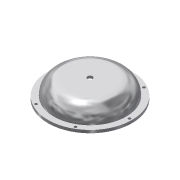
# Autodesk Inventor part: Kugel_oben_V5_Riza
Saved by Autodesk Inventor 2015 (Build 190159000, 159)
## iProperties
Created: 2015-06-19
Part Number: Kugel_oben_V5_Riza
Material: ABS-Kunststoff
Document SubType Name: Modeling
Designer: Johann
Density: 1.06 g/cm^3
Appearance: Aluminium - poliert
Mass: 35.3544 g
Surface Area: 192.96 cm^2
Volume: 33.3532 cm^3
Author: Johann
Autodesk Inventor part; units mm, degrees
ref_plane "YZ Plane" through (0, 0, 0) normal (1, 0, 0) x (0, 1, 0)
ref_plane "XZ Plane" through (0, 0, 0) normal (0, 1, 0) x (-1, 0, 0)
sketch "Skizze1" plane through (0, 0, 0) normal (1, 0, 0) x (0, 1, 0)
  line L0 (0, 0) -> (0, 55)
  line L1 (44, 0) -> (0, 0) construction
  line L2 (3.1, 21) -> (3.1, 18)
  line L3 (44, 0) -> (40, 0)
  line L4 (40, 0) -> (40, -5)
  line L5 (40, -5) -> (44, -5)
  line L6 (44, -5) -> (44, 0)
  line L7 (3.1, 18) -> (40, 18)
  line L8 (40, 18) -> (40, 0)
  line L9 (3.1, 21) -> (44, 21)
  line L10 (44, 21) -> (44, 0)
  point P0 (21.7075, 15.1998)
  dimension "d143" = 6.2
  dimension "d146" = 18
  dimension "d147" = 3
  dimension "d155" = 5
  dimension "d156" = 4
  dimension "d186" = 80
  constraints: 22 end point, 4 perpendicular, 3 horizontal, 3 vertical, 1 coincident, 1 point on line
  measures "d143" diameter of L2 L0
  measures "d146" distance from line of L1 L2.end
  measures "d147" distance of L2.start L2.end
  measures "d155" distance of L3.end L4.end
  measures "d156" distance of L1.start L3.end
  measures "d186" diameter of L8 L0
revolve "Umdrehung4" add sketch "Skizze1" angle 360 about axis through (0, 0, 0) along (0, 0, 1)
sketch "Skizze28" plane through (0, 0, -5) normal (0, 0, -1) x (-1, 0, 0)
  circle A0 centre (0, 0) radius 44 projected
  circle A1 centre (0, 0) radius 40 projected
  circle A2 centre (0, 0) radius 51
  dimension "d157" = 102
  constraints: 1 centre point, 1 coincident
  measures "d157" diameter of A2
extrude "Extrusion10" add sketch "Skizze28" against normal blind 7 contours A0 | A2
sketch "Skizze29" plane through (0, 0, -5) normal (0, 0, -1) x (-1, 0, 0)
  circle A0 centre (0, 0) radius 51 projected
  circle A1 centre (0, 0) radius 43
  dimension "d160" = 86
  constraints: 1 centre point
  measures "d160" diameter of A1
extrude "Extrusion11" cut sketch "Skizze29" against normal blind 3.5
sketch "Skizze30" plane through (0, 0, -1.5) normal (0, 0, -1) x (-1, 0, 0)
  circle A0 centre (0, 0) radius 43 projected
  circle A1 centre (0, 0) radius 51 projected
  point P0 (-48, 0)
  dimension "d163" = 48
  measures "d163" distance of point (0, 0) point (-48, 0)
hole "Bohrung3" at (48, 0, -1.5) direction (0, 0, 1) diameter 3.3 end through all
pattern_circular "Runde Anordnung2" count 6 over 360 about axis through (0, 0, -5) along (0, 0, 1) of "Bohrung3"
ref_plane "Arbeitsebene10" through (0, 0, 19) normal (0, 0, 1) x (1, 0, 0)
fillet "Rundung1" radius 15 1 edges at (0, -40, 18)
fillet "Rundung2" radius 18 1 edges at (0, -44, 21)
